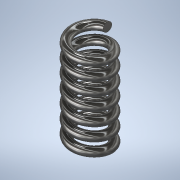
# Autodesk Inventor part: Coil_28
Saved by Autodesk Inventor 2021 (Build 250183000, 183)
## iProperties
Created: 2020-11-13
Part Number: Coil_28
Material: Liga de Nickel-Copper 400
Document SubType Name: Modeling
Designer: Lucas Moura
Density: 8.83 g/cm^3
Appearance: Cromado - Preto polido
Author: Lucas Moura
Autodesk Inventor part; units mm, degrees
ref_plane "YZ Plane" through (0, 0, 0) normal (1, 0, 0) x (0, 1, 0)
ref_plane "XZ Plane" through (0, 0, 0) normal (0, 1, 0) x (-1, 0, 0)
ref_plane "XY Plane" through (0, 0, 0) normal (0, 0, 1) x (1, 0, 0)
sketch "Sketch1" plane through (0, 0, 0) normal (1, 0, 0) x (0, 1, 0)
  line L0 (0, 0) -> (0, -0.2)
  circle A0 centre (0, -0.2) radius 0.05
  line L1 (0, 0) -> (3.06, 0)
  dimension "d0" = 0.2
  dimension "d1" = 0.1
  dimension "d2" = 3.06
  constraints: 4 end point, 1 centre point, 1 coincident, 1 horizontal, 1 vertical
  measures "d0" distance of L0.start L0.end
  measures "d1" diameter of A0
  measures "d2" distance of L0.start L1.end
coil "Coil1" sketch "Sketch1" operation add axis through (0, 0, 0) along (0, 1, 0) pitch 0.15 turns 7 hand left
body "Solid1"
